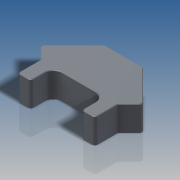
# Autodesk Inventor part: 99147-LtBluishGray
Saved by Autodesk Inventor 2016 SP2 (Build 200236200, 236)
## iProperties
Created: 2015-08-19
Part Number: 99147-LtBluishGray
Material: ABS Plastic
Document SubType Name: Modeling
Designer: D. Kohfeld
Mass: 0.954371 g
Surface Area: 6.84624 cm^2
Volume: 0.90035 cm^3
Density: 1.06 g/cm^3
Appearance: LtBluishGray
Author: D. Kohfeld
Autodesk Inventor part; units mm, degrees
ref_plane "YZ Plane" through (0, 0, 0) normal (1, 0, 0) x (0, 1, 0)
ref_plane "XZ Plane" through (0, 0, 0) normal (0, 1, 0) x (-1, 0, 0)
ref_plane "XY Plane" through (0, 0, 0) normal (0, 0, 1) x (1, 0, 0)
sketch "Sketch2" plane through (0, 0, 0) normal (0, 1, 0) x (-1, 0, 0)
  line L0 (-3.48, 2.7) -> (3.48, 2.7)
  arc A0 (3.48, 2.7) -> (5.28, 4.5) centre (3.48, 4.5) ccw
  line L1 (5.28, 4.5) -> (5.28, 7.38)
  line L2 (5.28, 7.38) -> (8, 7.38)
  line L3 (8, 7.38) -> (8, 2.62)
  line L4 (8, 2.62) -> (10.62, 0)
  line L5 (10.62, 0) -> (4, -6.62)
  line L6 (4, -6.62) -> (-4, -6.62)
  line L7 (-4, -6.62) -> (-10.62, 0)
  line L8 (-10.62, 0) -> (-8, 2.62)
  line L9 (-8, 2.62) -> (-8, 7.38)
  line L10 (-8, 7.38) -> (-5.28, 7.38)
  line L11 (-5.28, 7.38) -> (-5.28, 4.5)
  arc A1 (-5.28, 4.5) -> (-3.48, 2.7) centre (-3.48, 4.5) ccw
  point P0 (0, 0)
  point P1 (0, 2.7)
  point P2 (0, -6.62)
  dimension "d0" = 1.8
  dimension "d1" = 4.68
  dimension "d2" = 2.72
  dimension "d3" = 10.56
  dimension "d4" = 4.76
  dimension "d5" = 9.32
  dimension "d6" = 8
  constraints: 24 end point, 5 equal length, 4 horizontal, 4 point on circle, 4 tangent, 4 vertical, 3 perpendicular, 2 centre point, 2 horizontal alignment, 2 midpoint, 2 vertical alignment
  measures "d0" radius of A1
  measures "d1" distance between parallel lines of L10 L0
  measures "d2" distance between parallel lines of L11 L9
  measures "d3" distance between parallel lines of L1 L11
  measures "d4" distance from line of L3.end L2
  measures "d5" distance between parallel lines of L6 L0
  measures "d6" distance of L5.end L6.end
extrude "Extrusion1" add sketch "Sketch2" along normal mid plane 5.2
fillet "Fillet1" radius 0.6 6 edges at (-8, 0, 7.38) (-5.28, 0, 7.38) (5.28, 0, 7.38) (8, 0, 7.38) (10.62, 0, 0) (-10.62, 0, 0)
chamfer "Chamfer1" distance 0.12 angle 45 20 edges at (-8, 2.6, 4.7) (-7.8243, 2.6, 7.2043) (-6.64, 2.6, 7.38) (-5.4557, 2.6, 7.2043) (-5.28, 2.6, 5.64) (-4.7528, 2.6, 3.2272) (0, 2.6, 2.7) (4.7528, 2.6, 3.2272) (5.28, 2.6, 5.64) (5.4557, 2.6, 7.2043) (6.64, 2.6, 7.38) (7.8243, 2.6, 7.2043) (8, 2.6, 4.7) (-9.0979, 2.6, 1.5221) (-10.3715, 2.6, 0) (-7.0979, 2.6, -3.5221) (0, 2.6, -6.62) (7.0979, 2.6, -3.5221) (10.3715, 2.6, 0) (9.0979, 2.6, 1.5221)
equation "\"d6\" = lu"
equation "\"lu\" = 8"
body "Solid1"
